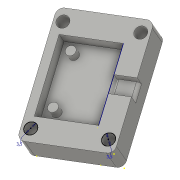
# Autodesk Inventor part: MPU6050_CASE_BOTTOM
Saved by Autodesk Inventor 2016 (Build 200138000, 138)
## iProperties
Created: 2015-05-21
Part Number: MPU6050_CASE_BOTTOM
Material: Generic
Document SubType Name: Modeling
Designer: Admin
Density: 1 g/cm^3
Appearance: Default
Author: Admin
Autodesk Inventor part; units mm, degrees
ref_plane "YZ Plane" through (0, 0, 0) normal (1, 0, 0) x (0, 1, 0)
ref_plane "XZ Plane" through (0, 0, 0) normal (0, 1, 0) x (-1, 0, 0)
ref_plane "XY Plane" through (0, 0, 0) normal (0, 0, 1) x (1, 0, 0)
sketch "Sketch1" plane through (0, 0, 0) normal (0, 1, 0) x (-1, 0, 0)
  point P0 (0, 0)
sketch "Sketch2" plane through (0, 0, 0) normal (0, 1, 0) x (-1, 0, 0)
  line L0 (0, 0) -> (35, 0)
  line L1 (35, 0) -> (35, 25)
  line L2 (35, 25) -> (0, 25)
  line L3 (0, 25) -> (0, 0)
  dimension "d0" = 35
  dimension "d1" = 25
  constraints: 8 end point, 2 parallel, 1 horizontal, 1 perpendicular
  measures "d0" distance of L2.end L1.end
  measures "d1" distance of L1.end L0.end
extrude "Extrusion1" add sketch "Sketch2" along normal blind 8
sketch "Sketch3" plane through (0, 8, 0) normal (0, 1, 0) x (1, 0, 0)
  line L0 (-28.1608, -22.5) -> (-6.6608, -22.5)
  line L1 (-6.6608, -22.5) -> (-6.6608, -6)
  line L2 (-6.6608, -6) -> (-28.1608, -6)
  line L3 (-28.1608, -6) -> (-28.1608, -22.5)
  dimension "d4" = 21.5
  dimension "d5" = 16.5
  constraints: 8 end point, 2 parallel, 1 horizontal, 1 perpendicular
  measures "d4" distance of L2.end L1.end
  measures "d5" distance of L1.end L0.end
extrude "Extrusion2" cut sketch "Sketch3" against normal blind 4
sketch "Sketch4" plane through (-6.6608, 8, 22.5) normal (0, 0, -1) x (-1, 0, 0)
  point P0 (-6.6608, -8)
sketch "Sketch5" plane through (-28.1608, 8, 6) normal (0, 0, 1) x (1, 0, 0)
  line L0 (0, -4) -> (21.5, -4)
  line L1 (21.5, -4) -> (21.5, 0)
  line L2 (21.5, 0) -> (0, 0)
  line L3 (0, 0) -> (0, -4)
  point P0 (28.1608, -8)
  constraints: 8 end point, 2 parallel, 1 horizontal, 1 perpendicular
sketch "Sketch12" plane through (0, 8, 0) normal (0, 1, 0) x (1, 0, 0)
  line L0 (-28.1608, -6) -> (-6.6608, -6) projected
  line L1 (0, 0) -> (-35, 0) projected
  line L2 (-15, -6) -> (-20, -6)
  line L3 (-20, -6) -> (-20, 0)
  line L4 (-20, 0) -> (-15, 0)
  line L5 (-15, 0) -> (-15, -6)
  dimension "d27" = 5
  constraints: 8 end point, 2 parallel, 2 point on line, 1 horizontal, 1 perpendicular
  measures "d27" distance of L3.end L4.end
extrude "Extrusion9" cut sketch "Sketch12" against normal blind 2.5
fillet "Fillet1" radius 2 1 edges at (-35, 4, 0)
fillet "Fillet2" radius 2 1 edges at (0, 4, 0)
fillet "Fillet3" radius 2 1 edges at (-35, 4, 25)
fillet "Fillet4" radius 2 1 edges at (0, 4, 25)
fillet "Fillet5" radius 0.5 1 edges at (-17.5, 5.5, 6)
sketch "Sketch13" plane through (0, 0, 0) normal (0, -1, 0) x (1, 0, 0)
  point P0 (0, 0)
sketch "Skizze18" plane through (0, 8, 0) normal (0, 1, 0) x (1, 0, 0)
  circle A0 centre (-3.5, -22.5) radius 1.75
  circle A1 centre (-3.5, -2.5) radius 1.75
  point P0 (0, 0)
  dimension "d47" = 3.5
  dimension "d48" = 3.5
  constraints: 2 centre point
  measures "d47" diameter of A0
  measures "d48" diameter of A1
extrude "Extrusion14" cut sketch "Skizze18" against normal blind 20 contours A0
extrude "Extrusion15" cut sketch "Skizze18" against normal blind 20 contours A1
sketch "Skizze19" plane through (0, 8, 0) normal (0, 1, 0) x (1, 0, 0)
  circle A0 centre (-31.5, -22.5) radius 1.75
  point P0 (0, 0)
  dimension "d53" = 3.5
  constraints: 1 centre point
  measures "d53" diameter of A0
extrude "Extrusion16" cut sketch "Skizze19" against normal blind 20
sketch "Skizze20" plane through (0, 8, 0) normal (0, 1, 0) x (1, 0, 0)
  circle A0 centre (-31.5, -2.5) radius 1.75
  point P0 (0, 0)
  dimension "d56" = 3.5
  constraints: 1 centre point
  measures "d56" diameter of A0
extrude "Extrusion17" cut sketch "Skizze20" against normal blind 20
sketch "Skizze21" plane through (0, 4, 0) normal (0, 1, 0) x (1, 0, 0)
  circle A0 centre (-10, -19) radius 1.5 projected
  circle A1 centre (-10, -19) radius 1.35
  point P0 (0, 0)
  dimension "d59" = 2.7
  constraints: 1 centre point, 1 coincident
  measures "d59" diameter of A1
extrude "Extrusion18" add sketch "Skizze21" along normal blind 3 contours A1
sketch "Skizze22" plane through (0, 4, 0) normal (0, 1, 0) x (1, 0, 0)
  circle A0 centre (-25, -19) radius 1.5 projected
  circle A1 centre (-25, -19) radius 1.35
  point P0 (0, 0)
  dimension "d62" = 2.7
  constraints: 1 centre point, 1 coincident
  measures "d62" diameter of A1
extrude "Extrusion19" add sketch "Skizze22" along normal blind 2.7 contours A1
fillet "Rundung6" radius 1 1 edges at (-17.5, 5.5, 0)
body "Solid1"
